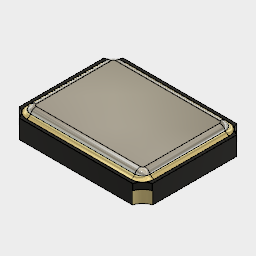
WiFi D1 MINI (Autodesk Fusion 360 archive; units mm, degrees)
design "2.5x3.2 quartz"
Autodesk Fusion 360 part; units mm, degrees
sketch "Sketch1" plane through (0, 0, 0) normal (0, 1, 0) x (1, 0, 0)
  line L0 (0, 0) -> (3.2, 0)
  line L1 (3.2, 0) -> (3.2, -2.5)
  line L2 (3.2, -2.5) -> (0, -2.5)
  line L3 (0, -2.5) -> (0, 0)
  dimension "d1" = 3.2
  dimension "d2" = 2.5
  measures "d1" distance of L0.start L0.end
  measures "d2" distance of L0.start L2.end
extrude "Extrude1" add sketch "Sketch1" along normal blind 0.45
sketch "Sketch2" plane through (0, 0.45, 0) normal (0, 1, 0) x (-1, 0, 0)
  line L0 (0, 2.5) -> (-3.2, 2.5)
  line L1 (-3.2, 2.5) -> (-3.2, 0)
  line L2 (-3.2, 0) -> (0, 0)
  line L3 (0, 0) -> (0, 2.5)
  circle A0 centre (0.1, -0.1) radius 0.35
  circle A1 centre (0.1, 2.6) radius 0.35
  circle A2 centre (-3.3, -0.1) radius 0.35
  circle A3 centre (-3.3, 2.6) radius 0.35
  arc A4 (0, 0.2354) -> (-0.2354, 0) centre (0.1, -0.1) ccw
  line L4 (0, 0.2354) -> (0, 2.2646)
  arc A5 (-0.2354, 2.5) -> (0, 2.2646) centre (0.1, 2.6) ccw
  line L5 (-0.2354, 2.5) -> (-2.9646, 2.5)
  arc A6 (-3.2, 2.2646) -> (-2.9646, 2.5) centre (-3.3, 2.6) ccw
  line L6 (-3.2, 2.2646) -> (-3.2, 0.2354)
  arc A7 (-2.9646, 0) -> (-3.2, 0.2354) centre (-3.3, -0.1) ccw
  line L7 (-2.9646, 0) -> (-0.2354, 0)
  arc A8 (0.2354, 0) -> (0, 0.2354) centre (-0.1, -0.1) ccw
  line L8 (0.2354, 0) -> (2.9646, 0)
  arc A9 (3.2, 0.2354) -> (2.9646, 0) centre (3.3, -0.1) ccw
  line L9 (3.2, 0.2354) -> (3.2, 2.2646)
  arc A10 (2.9646, 2.5) -> (3.2, 2.2646) centre (3.3, 2.6) ccw
  line L10 (2.9646, 2.5) -> (0.2354, 2.5)
  arc A11 (0, 2.2646) -> (0.2354, 2.5) centre (-0.1, 2.6) ccw
  line L11 (0, 2.2646) -> (0, 0.2354)
  arc A12 (0, 2.26) -> (0.24, 2.5) centre (-0.1, 2.6) ccw
  line L12 (0, 2.26) -> (0, 0.2354)
  arc A13 (0.2354, 0) -> (0, 0.2354) centre (-0.1, -0.1) ccw
  line L13 (0.2354, 0) -> (2.9646, 0)
  arc A14 (3.2, 0.2354) -> (2.9646, 0) centre (3.3, -0.1) ccw
  line L14 (3.2, 0.2354) -> (3.2, 2.2646)
  arc A15 (2.9646, 2.5) -> (3.2, 2.2646) centre (3.3, 2.6) ccw
  line L15 (2.9646, 2.5) -> (0.24, 2.5)
  dimension "d5" = 0.7
  dimension "d6" = 0.7
  dimension "d7" = 0.7
  dimension "d8" = 0.7
  measures "d5" diameter of A0
  measures "d6" diameter of A1
  measures "d7" diameter of A2
  measures "d8" diameter of A3
extrude "Extrude2" cut sketch "Sketch2" against normal blind 0.45 contours L0 L1 A3 A6
extrude "Extrude3" cut sketch "Sketch2" against normal blind 0.45 contours L1 L2 A2 A7
extrude "Extrude4" cut sketch "Sketch2" against normal blind 0.45 contours L0 L3 A1 A5
extrude "Extrude5" cut sketch "Sketch2" against normal blind 0.45 contours L2 L3 A0 A4
sketch "Sketch3" plane through (0, 0.45, 0) normal (0, 1, 0) x (-1, 0, 0)
  arc A0 (0, 0.2354) -> (-0.2354, 0) centre (0.1, -0.1) ccw
  line L0 (0, 0.2354) -> (0, 2.2646)
  arc A1 (-0.2354, 2.5) -> (0, 2.2646) centre (0.1, 2.6) ccw
  line L1 (-0.2354, 2.5) -> (-2.9646, 2.5)
  arc A2 (-3.2, 2.2646) -> (-2.9646, 2.5) centre (-3.3, 2.6) ccw
  line L2 (-3.2, 2.2646) -> (-3.2, 0.2354)
  arc A3 (-2.9646, 0) -> (-3.2, 0.2354) centre (-3.3, -0.1) ccw
  line L3 (-2.9646, 0) -> (-0.2354, 0)
  line L4 (-0.3475, 2.3525) -> (-2.8525, 2.3525)
  line L5 (-3.0525, 2.1525) -> (-3.0525, 0.3475)
  line L6 (-2.8525, 0.1475) -> (-0.3475, 0.1475)
  line L7 (-0.1475, 0.3475) -> (-0.1475, 2.1525)
  arc A4 (-0.3475, 0.1475) -> (-0.1475, 0.3475) centre (-0.3475, 0.3475) ccw
  arc A5 (-0.1475, 2.1525) -> (-0.3475, 2.3525) centre (-0.3475, 2.1525) ccw
  arc A6 (-3.0525, 0.3475) -> (-2.8525, 0.1475) centre (-2.8525, 0.3475) ccw
  arc A7 (-2.8525, 2.3525) -> (-3.0525, 2.1525) centre (-2.8525, 2.1525) ccw
  dimension "d17" = 0.2
  measures "d17" radius of A4
extrude "Extrude6" add sketch "Sketch3" along normal blind 0.15 contours L4 L5 L6 L7 A4 A5 A6 A7
fillet "Fillet1" radius 0.15 8 edges at (1.6, 0.6, 2.3525) (2.9939, 0.6, 2.2939) (3.0525, 0.6, 1.25) (2.9939, 0.6, 0.2061) (1.6, 0.6, 0.1475) (0.2061, 0.6, 0.2061) (0.1475, 0.6, 1.25) (0.2061, 0.6, 2.2939)
fillet "Fillet2" radius 0.1 8 edges at (0.1475, 0.45, 1.25) (0.2061, 0.45, 0.2061) (1.6, 0.45, 0.1475) (2.9939, 0.45, 0.2061) (3.0525, 0.45, 1.25) (2.9939, 0.45, 2.2939) (1.6, 0.45, 2.3525) (0.2061, 0.45, 2.2939)
sketch "Sketch4" plane through (0, 0, 0) normal (0, -1, 0) x (1, 0, 0)
  arc A0 (0.2354, 0) -> (0, 0.2354) centre (-0.1, -0.1) ccw
  line L0 (0.2354, 0) -> (2.9646, 0)
  arc A1 (3.2, 0.2354) -> (2.9646, 0) centre (3.3, -0.1) ccw
  line L1 (3.2, 0.2354) -> (3.2, 2.2646)
  arc A2 (2.9646, 2.5) -> (3.2, 2.2646) centre (3.3, 2.6) ccw
  line L2 (2.9646, 2.5) -> (0.2354, 2.5)
  arc A3 (0, 2.2646) -> (0.2354, 2.5) centre (-0.1, 2.6) ccw
  line L3 (0, 2.2646) -> (0, 0.2354)
  arc A4 (0, 2.26) -> (0.24, 2.5) centre (-0.1, 2.6) ccw
extrude "Extrude7" cut sketch "Sketch4" against normal blind 0.3 contours L2 A3 L3 A4
sketch "Sketch5" plane through (0, 0, 0) normal (0, 1, 0) x (1, 0, 0)
sketch "Sketch6" plane through (0, 0, 0) normal (0, -1, 0) x (1, 0, 0)
  arc A0 (0, 2.26) -> (0.24, 2.5) centre (-0.1, 2.6) ccw
  line L0 (0, 2.26) -> (0, 0.2354)
  arc A1 (0.2354, 0) -> (0, 0.2354) centre (-0.1, -0.1) ccw
  line L1 (0.2354, 0) -> (2.9646, 0)
  arc A2 (3.2, 0.2354) -> (2.9646, 0) centre (3.3, -0.1) ccw
  line L2 (3.2, 0.2354) -> (3.2, 2.2646)
  arc A3 (2.9646, 2.5) -> (3.2, 2.2646) centre (3.3, 2.6) ccw
  line L3 (2.9646, 2.5) -> (0.24, 2.5)
  arc A4 (0.2455, 0) -> (0, 0.2455) centre (-0.1, -0.1) ccw
  arc A5 (2.9552, 2.5) -> (3.2, 2.2552) centre (3.3, 2.6) ccw
  arc A6 (3.2, 0.2434) -> (2.9566, 0) centre (3.3, -0.1) ccw
extrude "Extrude8" cut sketch "Sketch6" against normal blind 0.3 contours L0 A1 L1 A4 | L2 A3 L3 A5 | L1 A2 L2 A6
